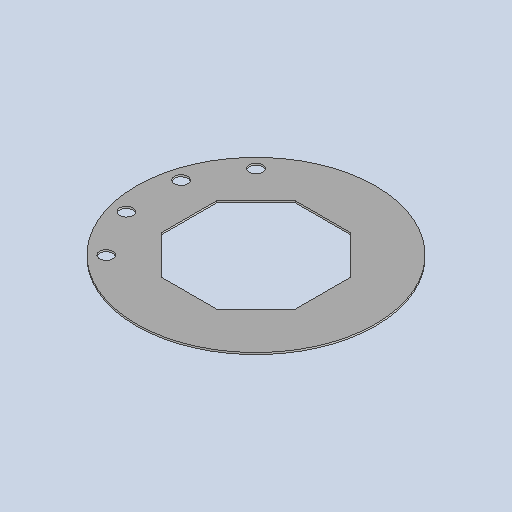
# Autodesk Inventor part: KND-9651 DrSysB MAIN FLANGE 01
Saved by Autodesk Inventor 2026.2 (Build 302298000, 298)
## iProperties
Created: 2025-06-24
Part Number: KND-9651 DrSysB MAIN FLANGE 01
Material: Stainless Steel
Document SubType Name: Sheet Metal
Designer: admin
Mass: 326.359 g
Surface Area: 301.648 cm^2
Volume: 40.7948 cm^3
Density: 8 g/cm^3
Flat Pattern Width: 39.5 cm
Flat Pattern Length: 39.5 cm
Flat Pattern Area: 1560.25 cm^2
Sheet Metal Rule: Default
Sheet Metal Width: 395,000 mm
Sheet Metal Length: 395,000 mm
Sheet Metal Area: 156025,000 mm^2
Appearance: Default
Author: user
Autodesk Inventor part; units mm, degrees
ref_plane "YZ Plane" through (0, 0, 0) normal (1, 0, 0) x (0, 1, 0)
ref_plane "XZ Plane" through (0, 0, 0) normal (0, 1, 0) x (-1, 0, 0)
ref_plane "XY Plane" through (0, 0, 0) normal (0, 0, 1) x (1, 0, 0)
sketch "Sketch1" plane through (0, 0, 0) normal (0, 0, 1) x (1, 0, 0)
  circle A0 centre (0, 0) radius 197.5
  circle A1 centre (-123.7437, 123.7437) radius 11
  circle A2 centre (0, 0) radius 175 construction
  circle A3 centre (-169.037, 45.2933) radius 11
  circle A4 centre (-169.037, -45.2933) radius 11
  circle A5 centre (-123.7437, -123.7437) radius 11
  line L0 (45.5635, -110) -> (-45.5635, -110)
  line L1 (-45.5635, -110) -> (-110, -45.5635)
  line L2 (-110, -45.5635) -> (-110, 45.5635)
  line L3 (-110, 45.5635) -> (-45.5635, 110)
  line L4 (-45.5635, 110) -> (45.5635, 110)
  line L5 (45.5635, 110) -> (110, 45.5635)
  line L6 (110, 45.5635) -> (110, -45.5635)
  line L7 (110, -45.5635) -> (45.5635, -110)
  line L8 (0, 0) -> (-77.7817, 77.7817) construction
  circle A6 centre (-45.2933, -169.037) radius 11
  circle A7 centre (45.2933, -169.037) radius 11
  circle A8 centre (123.7437, -123.7437) radius 11
  circle A9 centre (169.037, -45.2933) radius 11
  circle A10 centre (169.037, 45.2933) radius 11
  circle A11 centre (123.7437, 123.7437) radius 11
  circle A12 centre (45.2933, 169.037) radius 11
  circle A13 centre (-45.2933, 169.037) radius 11
  dimension "d171" = 350
  dimension "d157" = 395
  dimension "d170" = 22
  dimension "d174" = 360
  dimension "d176" = 220
  measures "d157" diameter of A0
  measures "d170" diameter of A1
  measures "d176" distance between parallel lines of L4 L0
extrude "Plate5" add sketch "Sketch1" along normal blind 3 contours A0 | A6 | A7 | A8 | A9 | A10 | A11 | A12 | A13
derived "KND-1401 DrSysB DIMentions 01.ipt"
body "Solid3"
